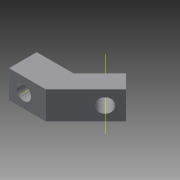
# Autodesk Inventor part: connect stepper
Saved by Autodesk Inventor 2013 (Build 170138000, 138)
## iProperties
Created: 2013-01-04
Part Number: connect stepper
Material: Generic
Document SubType Name: Modeling
Designer: Nico
Density: 1 g/cm^3
Author: Nico
Autodesk Inventor part; units mm, degrees
ref_plane "YZ Plane" through (0, 0, 0) normal (1, 0, 0) x (0, 1, 0)
ref_plane "XZ Plane" through (0, 0, 0) normal (0, 1, 0) x (-1, 0, 0)
ref_plane "XY Plane" through (0, 0, 0) normal (0, 0, 1) x (1, 0, 0)
sketch "Sketch1" plane through (0, 0, 0) normal (0, 0, 1) x (1, 0, 0)
  line L0 (0, 0) -> (20, 0)
  line L1 (20, 0) -> (20, 15)
  line L2 (20, 15) -> (0, 15)
  line L3 (0, 15) -> (0, 0)
  dimension "d0" = 20
  dimension "d1" = 15
  constraints: 8 end point, 2 parallel, 1 horizontal, 1 perpendicular
  measures "d0" distance of L0.start L0.end
  measures "d1" distance of L2.end L0.start
extrude "Extrusion1" add sketch "Sketch1" along normal blind 15
sketch "Sketch2" plane through (0, 15, 0) normal (0, 1, 0) x (1, 0, 0)
  line L0 (0, 0) -> (0, -15) projected
  circle A0 centre (8, -7.5) radius 3.9
  dimension "d4" = 7.8
  dimension "d6" = 8
  constraints: 1 centre point
  measures "d4" diameter of A0
  measures "d6" distance from line of A0.centre L0
extrude "Extrusion2" cut sketch "Sketch2" against normal blind 15
sketch "Sketch3" plane through (0, 0, 15) normal (0, 0, 1) x (1, 0, 0)
  line L0 (0, 0) -> (20, 0) projected
  line L1 (20, 0) -> (20, 15) projected
  line L2 (20, 0) -> (34.1421, 14.1421)
  line L3 (20, 15) -> (34.1421, 29.1421)
  line L4 (34.1421, 14.1421) -> (41.6421, 21.6421)
  line L5 (41.6421, 21.6421) -> (34.1421, 29.1421)
  dimension "d9" = 45
  dimension "d10" = 20
  dimension "d11" = 20
  constraints: 8 end point, 2 parallel, 1 perpendicular
  measures "d9" angle of L0 L2
  measures "d10" distance of L0.end L2.end
  measures "d11" distance of L1.end L3.end
extrude "Extrusion3" add sketch "Sketch3" against normal blind 15
sketch "Sketch4" plane through (34.1421, 29.1421, 15) normal (-0.7071, 0.7071, 0) x (0.7071, 0.7071, 0)
  line L0 (0, 0) -> (0, 15) projected
  circle A0 centre (-8, 7.5) radius 3.9
  point P0 (-44.7487, 15)
  dimension "d14" = 7.8
  dimension "d16" = 8
  constraints: 1 centre point
  measures "d14" diameter of A0
  measures "d16" distance from line of A0.centre L0
extrude "Extrusion4" cut sketch "Sketch4" against normal blind 15
body "Solid1"
